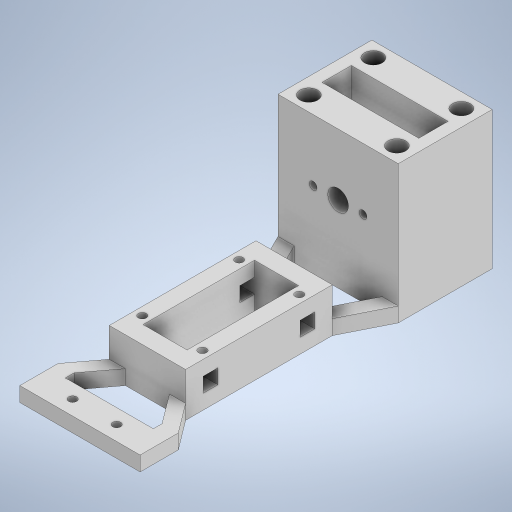
# Autodesk Inventor part: Houder encodere
Saved by Autodesk Inventor 2023.2 (Build 272271030, 271C)
## iProperties
Created: 2023-03-09
Part Number: Houder encodere
Material: Generic
Document SubType Name: Modeling
Designer: daanj
Density: 1 g/cm^3
Appearance: Default
Author: daanj
Autodesk Inventor part; units mm, degrees
ref_plane "YZ Plane" through (0, 0, 0) normal (1, 0, 0) x (0, 1, 0)
ref_plane "XZ Plane" through (0, 0, 0) normal (0, 1, 0) x (-1, 0, 0)
ref_plane "XY Plane" through (0, 0, 0) normal (0, 0, 1) x (1, 0, 0)
sketch "Sketch1" plane through (0, 0, 0) normal (0, 1, 0) x (-1, 0, 0)
  line L0 (20.5, -60) -> (-20.5, -60)
  line L1 (-20.5, -60) -> (-20.5, 60)
  line L2 (-20.5, 60) -> (20.5, 60)
  line L3 (20.5, -60) -> (-20.5, 60) construction
  line L4 (-20.5, -60) -> (20.5, 60) construction
  circle A0 centre (7.5, 55) radius 1.35
  circle A1 centre (-7.5, 55) radius 1.35
  circle A2 centre (15, -33) radius 1.35
  circle A3 centre (15, -55) radius 1.35
  circle A4 centre (-15, -55) radius 1.35
  circle A5 centre (-15, -33) radius 1.35
  line L5 (-13, -13) -> (-13, 37)
  line L6 (13, 37) -> (13, -13)
  line L7 (20.5, -33) -> (20.5, -28)
  line L8 (20.5, -28) -> (13, -13)
  line L9 (-13, -13) -> (-20.5, -28)
  line L10 (20.5, 55) -> (20.5, 54)
  line L11 (20.5, 47) -> (13, 37)
  line L12 (-13, 37) -> (-20.5, 47)
  line L13 (20.5, 60) -> (20.5, 47)
  line L14 (20.5, -28) -> (20.5, -60)
  line L15 (16.5, -49) -> (-16.5, -49)
  line L16 (-16.5, -49) -> (-16.5, -39)
  line L17 (-16.5, -39) -> (16.5, -39)
  line L18 (16.5, -39) -> (16.5, -49)
  line L19 (15, -28) -> (-15, -28)
  line L20 (-15, -28) -> (-7.5, -13)
  line L21 (-7.5, -13) -> (7.5, -13)
  line L22 (7.5, -13) -> (15, -28)
  line L23 (7.5, -7) -> (-7.5, -7)
  line L24 (-7.5, -7) -> (-7.5, 31)
  line L25 (-7.5, 31) -> (7.5, 31)
  line L26 (7.5, 31) -> (7.5, -7)
  line L27 (7.5, 37) -> (-7.5, 37)
  line L28 (-7.5, 37) -> (-15, 47)
  line L29 (7.5, 37) -> (15, 47)
  line L30 (15, 47) -> (15, 50)
  line L31 (15, 50) -> (-15, 50)
  line L32 (-15, 50) -> (-15, 47)
  point P0 (0, 0)
  dimension "d0" = 41
  dimension "d1" = 120
  dimension "d2" = 5
  dimension "d3" = 2.7
  dimension "d5" = 22
  dimension "d6" = 15
  dimension "d7" = 7.5
  dimension "d8" = 30
  dimension "d9" = 15
  dimension "d10" = 88
  dimension "d11" = 50
  dimension "d12" = 26
  dimension "d14" = 13
  dimension "d15" = 5
  dimension "d16" = 8
  dimension "d17" = 33
  dimension "d18" = 16.5
  dimension "d19" = 10
  dimension "d20" = 6
  dimension "d21" = 5
  dimension "d22" = 15
  dimension "d23" = 6
  dimension "d25" = 6
  dimension "d28" = 5.5
  dimension "d29" = 5.5
  dimension "d30" = 5
  dimension "d33" = 0
  dimension "d34" = 5.5
  dimension "d35" = 5.5
  constraints: 66 end point, 9 parallel, 6 centre point, 5 equal radius, 5 horizontal, 5 perpendicular, 5 point on line, 3 horizontal alignment, 2 midpoint, 2 vertical alignment, 1 vertical
  measures "d0" distance of L0.start L0.end
  measures "d1" distance of L0.end L1.end
  measures "d2" distance from line of L2 A0.centre
  measures "d3" diameter of A0
  measures "d5" distance of A3.centre A2.centre
  measures "d6" distance of A1.centre A0.centre
  measures "d7" horizontal distance of point (0, 0) A0.centre
  measures "d8" distance of A5.centre A2.centre
  measures "d9" horizontal distance of point (0, 0) A2.centre
  measures "d10" vertical distance of A0.centre A2.centre
  measures "d11" distance of L5.start L5.end
  measures "d12" distance of L6.end L5.start
  measures "d14" distance from line of point (0, 0) L5
  measures "d15" distance of L7.start L7.end
  measures "d16" distance of L10.start L11.start
  measures "d17" distance of L15.start L15.end
  measures "d18" distance from line of point (0, 0) L18
  measures "d19" distance of L17.end L15.start
  measures "d20" distance from line of A3.centre L15
  measures "d21" distance of A2.centre L19.start
  measures "d22" distance of L20.end L21.end
  measures "d23" distance between parallel lines of L21 L23
  measures "d25" distance from line of L25 L6.start
  measures "d28" distance of L27.start L6.start
  measures "d29" distance of L12.end L28.end
  measures "d30" distance from line of L31 A0.centre
  measures "d33" vertical distance of L21.end L6.end
  measures "d34" distance of L6.end L21.end
  measures "d35" distance of L5.start L20.end
extrude "Extrusion1" add sketch "Sketch1" along normal blind 5 contours L0 L1 L9 L5 L12 L2 L13 L10 L11 L6 L8 L7 L14
sketch "Sketch2" plane through (0, 5, 0) normal (0, 1, 0) x (1, 0, 0)
  line L0 (-20.5, 60) -> (-20.5, 28) projected
  line L1 (-7.5, 13) -> (-15, 28) projected
  line L2 (-20.5, 28) -> (-15, 28)
  line L3 (15, 28) -> (7.5, 13) projected
  line L4 (13, 13) -> (20.5, 28) projected
  line L5 (15, 28) -> (20.5, 28)
  line L6 (20.5, 60) -> (-20.5, 60) projected
  line L7 (20.5, 28) -> (20.5, 60) projected
  line L8 (16.5, 39) -> (-16.5, 39) projected
  line L9 (-15, 28) -> (15, 28) projected
  circle A0 centre (-15, 33) radius 1.35 projected
  circle A1 centre (15, 33) radius 1.35 projected
  line L10 (-16.5, 49) -> (16.5, 49) projected
  line L11 (-16.5, 39) -> (-16.5, 49) projected
  line L12 (16.5, 49) -> (16.5, 39) projected
  circle A2 centre (15, 55) radius 1.35 projected
  circle A3 centre (-15, 55) radius 1.35 projected
  circle A4 centre (-15, 55) radius 3
  circle A5 centre (15, 55) radius 3
  circle A6 centre (15, 33) radius 3
  circle A7 centre (-15, 33) radius 3
  point P0 (0, 0)
  dimension "d36" = 6
  dimension "d37" = 6
  dimension "d38" = 6
  dimension "d39" = 6
  constraints: 4 centre point, 4 coincident, 4 end point, 2 horizontal
  measures "d36" diameter of A4
  measures "d37" diameter of A5
  measures "d38" diameter of A6
  measures "d39" diameter of A7
extrude "Extrusion2" add sketch "Sketch2" along normal blind 42 contours L6 L7 L5 L9 L2 L0
sketch "Sketch3" plane through (-15, 0, -28) normal (0, 0, 1) x (1, 0, 0)
  line L0 (-5.5, 5) -> (-5.5, 47) projected
  line L1 (-5.5, 47) -> (35.5, 47) projected
  point P0 (15, 0)
  point P1 (15, 26)
  dimension "d42" = 20.5
  dimension "d43" = 21
  measures "d42" distance from line of L0 point (15, 26)
  measures "d43" distance from line of L1 point (15, 26)
hole "Hole1" at (0, 26, -28) direction (0, 0, -1) diameter 7 end through all
sketch "Sketch4" plane through (0, 5, 0) normal (0, 1, 0) x (1, 0, 0)
  line L0 (-7.5, -31) -> (-7.5, 7) projected
  line L1 (7.5, 7) -> (7.5, -31) projected
  line L2 (-7.5, 7) -> (7.5, 7) projected
  line L3 (7.5, -31) -> (-7.5, -31) projected
  line L4 (13, -37) -> (13, 13) projected
  line L5 (-13, 13) -> (13, 13)
  line L6 (13, 13) -> (13, -37)
  line L7 (13, -37) -> (-13, -37)
  line L8 (-13, -37) -> (-13, 13)
  circle A0 centre (-10.25, 4.5) radius 1.35
  circle A1 centre (-10.25, -28.5) radius 1.35
  circle A2 centre (10.25, -28.5) radius 1.35
  circle A3 centre (10.25, 4.5) radius 1.35
  point P0 (0, 0)
  dimension "d63" = 2.7
  dimension "d64" = 2.5
  dimension "d65" = 2.5
  dimension "d66" = 2.75
  dimension "d67" = 2.75
  constraints: 8 end point, 4 centre point, 3 equal radius, 2 horizontal alignment, 2 parallel, 2 vertical alignment, 1 horizontal, 1 perpendicular
  measures "d63" diameter of A3
  measures "d64" vertical distance of L1.start A3.centre
  measures "d65" vertical distance of L1.end A2.centre
  measures "d66" distance from line of L4 A3.centre
  measures "d67" distance from line of L8 A0.centre
extrude "Extrusion5" add sketch "Sketch4" along normal blind 10
sketch "Sketch5" plane through (-13, 0, -13) normal (-1, 0, 0) x (0, 0, 1)
  line L0 (0, 0) -> (0, 5) construction
  line L1 (60, 5) -> (50, 5) construction
  line L2 (6, 5) -> (11, 5)
  line L3 (11, 5) -> (11, 10)
  line L4 (11, 10) -> (6, 10)
  line L5 (6, 10) -> (6, 5)
  line L6 (44, 5) -> (39, 5)
  line L7 (39, 5) -> (39, 10)
  line L8 (39, 10) -> (44, 10)
  line L9 (44, 10) -> (44, 5)
  point P0 (13, 0)
  dimension "d53" = 5
  dimension "d54" = 5
  dimension "d55" = 0
  dimension "d56" = 5
  dimension "d57" = 5
  dimension "d58" = 6
  dimension "d59" = 6
  dimension "d60" = 5
  constraints: 16 end point, 4 parallel, 2 horizontal, 2 perpendicular, 1 point on line
  measures "d53" distance of L3.end L4.end
  measures "d54" distance of L2.end L3.end
  measures "d55" distance from line of L0.end L2
  measures "d56" distance of L6.start L6.end
  measures "d57" distance of L7.end L8.end
  measures "d58" distance from line of L9 L1.end
  measures "d59" distance from line of L0.end L5
  measures "d60" distance of L6.end L7.end
extrude "Extrusion4" cut sketch "Sketch5" against normal through all
sketch "Sketch6" plane through (-15, 0, -28) normal (0, 0, 1) x (1, 0, 0)
  circle A0 centre (15, 26) radius 3.5 projected
  circle A1 centre (15, 26) radius 8.5 construction
  line L0 (15, 26) -> (25.2915, 26) construction
  line L1 (27, 47) -> (27, 5) construction
  line L2 (25.2915, 26) -> (5.5322, 26) construction
  circle A2 centre (23.5, 26) radius 1.3
  circle A3 centre (6.5, 26) radius 1.3
  point P0 (15, 0)
  dimension "d70" = 17
  dimension "d71" = 2.6
  dimension "d72" = 2.6
  constraints: 4 end point, 3 centre point, 3 point on line, 2 point on circle, 1 coincident, 1 perpendicular
  measures "d70" diameter of A1
  measures "d71" diameter of A2
  measures "d72" diameter of A3
extrude "Extrusion6" cut sketch "Sketch6" against normal blind 10 contours A2 | A3
body "Solid1"
